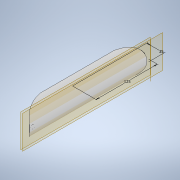
# Autodesk Inventor part: Deckel_Parachute_2
Saved by Autodesk Inventor 2020 (Build 240168000, 168)
## iProperties
Created: 2022-01-25
Part Number: Deckel_Parachute_2
Material: Generisch
Document SubType Name: Modeling
Designer: sp
Density: 1 g/cm^3
Appearance: Vorgabe
Author: sp
Autodesk Inventor part; units mm, degrees
ref_plane "XY Plane" through (0, 0, 0) normal (0, 0, 1) x (1, 0, 0)
sketch "Skizze1" plane through (0, 0, 0) normal (0, 0, 1) x (1, 0, 0)
  circle A0 centre (0, 0) radius 32
  circle A1 centre (0, 0) radius 30
  dimension "d0" = 64
  dimension "d1" = 60
  constraints: 2 centre point, 2 coincident
  measures "d0" diameter of A0
  measures "d1" diameter of A1
extrude "Extrusion1" add sketch "Skizze1" along normal mid plane 300
sketch "Skizze2" plane through (0, 0, 0) normal (0, 1, 0) x (-1, 0, 0)
  line L0 (-10, 169.5773) -> (-10, -169.8146) construction
  line L1 (-74.8376, 0) -> (82.6362, 0) construction
  line L2 (-10, 75) -> (-10, -75)
  line L3 (-32, -150) -> (-32, 150) projected
  line L4 (32, 150) -> (-32, 150) projected
  line L5 (-32, -150) -> (32, -150) projected
  spline S0 degree 2 poles (-10, 75) (-19.6473, 135.9655) (-72.8449, 128.3193) knots 0 0 0 1 1 1
  spline S1 degree 2 poles (-10, -75) (-19.4526, -135.7499) (-74.8376, -130) knots 0 0 0 1 1 1
  line L6 (-72.8449, 128.3193) -> (-74.8376, -130)
  line L7 (-32, 120) -> (-32, 150)
  line L8 (-32, 150) -> (32, 150)
  line L9 (32, 150) -> (32, -150)
  line L10 (32, -150) -> (32, 150) projected
  line L11 (32, -150) -> (-32, -150)
  line L12 (-32, -150) -> (-32, -120)
  point P0 (0, 0)
  dimension "d4" = 10
  dimension "d5" = 150
  dimension "d6" = 30
  dimension "d7" = 30
  constraints: 18 end point, 5 point on line, 3 perpendicular, 2 collinear, 1 horizontal, 1 symmetric about line, 1 vertical, 6 other
  measures "d4" distance from line of point (0, 0) L0
  measures "d5" distance of L2.start L2.end
  measures "d6" distance from line of L7.start L4
  measures "d7" distance from line of L12.end L5
extrude "Extrusion3" cut sketch "Skizze2" along normal mid plane 100 contours S0 L3 L4 L9 L5 S1 L2
ref_plane "Arbeitsebene1" through (26.5, 0, 0) normal (1, 0, 0) x (0, 1, 0)
sketch "Skizze3" plane through (26.5, 0, 0) normal (1, 0, 0) x (0, 1, 0)
  line L0 (0, 187.9338) -> (0, -197.3783) construction
  line L1 (-84.909, 0) -> (82.6972, 0) construction
  circle A0 centre (0, 113) radius 4
  point P0 (0, 0)
  dimension "d13" = 8
  dimension "d14" = 113
  constraints: 4 end point, 3 point on line, 1 centre point, 1 horizontal, 1 vertical
  measures "d13" diameter of A0
  measures "d14" distance of point (0, 0) A0.centre
extrude "Extrusion4" cut sketch "Skizze3" along normal blind 5
sketch "Skizze4" plane through (0, 0, 0) normal (0, 1, 0) x (-1, 0, 0)
  point P0 (0, 0)
  point P1 (-35, -125)
  dimension "d17" = 125
  dimension "d18" = 35
  measures "d17" vertical distance of point (-35, -125) point (0, 0)
  measures "d18" horizontal distance of point (0, 0) point (-35, -125)
ref_plane "Arbeitsebene2" through (31, 0, 0) normal (1, 0, 0) x (0, 1, 0)
sketch "Skizze5" plane through (31, 0, 0) normal (1, 0, 0) x (0, 1, 0)
  line L0 (-5, -105) -> (5, -105)
  line L1 (5, -105) -> (5, -115)
  line L2 (5, -115) -> (-5, -115)
  line L3 (-5, -115) -> (-5, -105)
  line L4 (-90.4877, 0) -> (95.944, 0) construction
  line L5 (0, -287.2342) -> (0, 33.44) construction
  line L6 (-127.7741, -125) -> (133.2304, -125) projected
  point P0 (0, 0)
  dimension "d20" = 10
  dimension "d21" = 105
  dimension "d22" = 10
  constraints: 12 end point, 2 horizontal, 2 parallel, 2 point on line, 1 perpendicular, 1 vertical, 1 other
  measures "d20" distance of L1.end L2.end
  measures "d21" distance between parallel lines of L4 L0
  measures "d22" distance of L2.end L0.start
revolve "Umdrehung1" add sketch "Skizze5" angle 100 about axis through (31, 0, -125) along (0, -1, 0)
